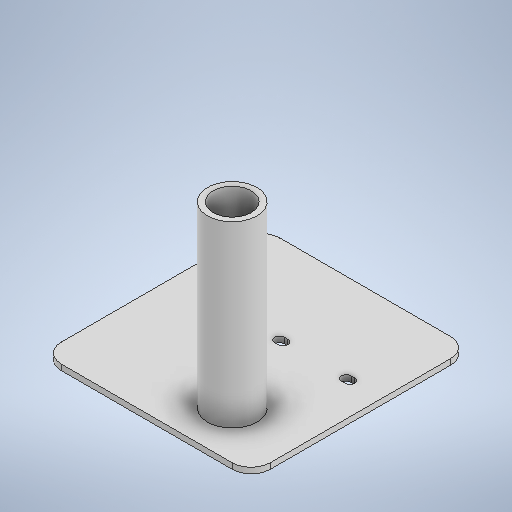
# Autodesk Inventor part: TopMount
Saved by Autodesk Inventor 2025.2 (Build 292293000, 293)
## iProperties
Created: 2025-07-18
Part Number: TopMount
Material: Generic
Document SubType Name: Modeling
Designer: Simon
Density: 1 g/cm^3
Appearance: Default
Author: Simon
Autodesk Inventor part; units mm, degrees
ref_plane "YZ Plane" through (0, 0, 0) normal (1, 0, 0) x (0, 1, 0)
ref_plane "XZ Plane" through (0, 0, 0) normal (0, 1, 0) x (-1, 0, 0)
ref_plane "XY Plane" through (0, 0, 0) normal (0, 0, 1) x (1, 0, 0)
sketch "Sketch1" plane through (0, 0, 0) normal (0, 1, 0) x (-1, 0, 0)
  line L0 (-75, 47.5) -> (75, 47.5)
  line L1 (75, 47.5) -> (75, -47.5)
  line L2 (75, -47.5) -> (-75, -47.5)
  line L3 (-75, -47.5) -> (-75, 47.5)
  line L4 (-75, 47.5) -> (75, -47.5) construction
  line L5 (75, 47.5) -> (-75, -47.5) construction
  point P0 (0, 0)
  dimension "d0" = 150
  dimension "d1" = 95
  constraints: 12 end point, 2 midpoint, 2 parallel, 1 horizontal, 1 perpendicular
  measures "d0" distance of L1.end L2.end
  measures "d1" distance of L0.end L1.end
extrude "Extrusion1" add sketch "Sketch1" along normal blind 3
sketch "Sketch6" plane through (0, 3, 0) normal (0, 1, 0) x (1, 0, 0)
  line L0 (75, 47.5) -> (-75, 47.5) projected
  line L1 (0, 47.5) -> (0, 22.5)
  line L2 (0, 22.5) -> (0, -20.7)
  line L3 (0, -20.7) -> (0, 0.9)
  line L4 (0, 0.9) -> (-53.4, 0.9)
  line L5 (-18.65, 0.9) -> (18.65, 0.9)
  circle A0 centre (18.65, 0.9) radius 2.5
  circle A1 centre (-18.65, 0.9) radius 2.5
  line L6 (-18.65, 0.9) -> (-16.65, 0.9)
  line L7 (18.65, 0.9) -> (16.65, 0.9)
  circle A2 centre (16.65, 0.9) radius 2.5
  circle A3 centre (-16.65, 0.9) radius 2.5
  line L8 (-18.65, 3.4) -> (-16.65, 3.4)
  line L9 (-18.65, -1.6) -> (-16.65, -1.6)
  line L10 (16.65, 3.4) -> (18.65, 3.4)
  line L11 (16.65, -1.6) -> (18.65, -1.6)
  point P0 (0, 0)
  dimension "d40" = 25
  dimension "d41" = 43.2
  dimension "d42" = 53.4
  dimension "d46" = 37.3
  dimension "d47" = 5
  dimension "d48" = 5
  dimension "d49" = 2
  dimension "d50" = 2
  dimension "d51" = 5
  dimension "d52" = 5
  constraints: 22 end point, 8 point on circle, 8 tangent, 4 centre point, 4 coincident, 3 midpoint, 3 point on line, 1 horizontal, 1 perpendicular, 1 vertical
  measures "d40" distance of L1.start L1.end
  measures "d41" distance of L1.end L2.end
  measures "d42" distance of L3.end L4.end
  measures "d46" distance of L5.start L5.end
  measures "d47" diameter of A0
  measures "d48" diameter of A1
  measures "d49" distance of L6.start L6.end
  measures "d50" distance of L7.start L7.end
  measures "d51" diameter of A2
  measures "d52" diameter of A3
extrude "Extrusion6" cut sketch "Sketch6" against normal through all
sketch "Sketch7" plane through (0, 3, 0) normal (0, 1, 0) x (1, 0, 0)
  line L0 (75, 47.5) -> (-75, 47.5) projected
  line L1 (-75, -47.5) -> (75, -47.5) projected
  line L2 (75, 47.5) -> (35, 47.5)
  line L3 (35, 47.5) -> (35, -47.5)
  line L4 (35, -47.5) -> (75, -47.5)
  line L5 (75, -47.5) -> (75, 47.5)
  point P0 (0, 0)
  point P1 (75, -47.5)
  dimension "d55" = 40
  constraints: 8 end point, 2 parallel, 1 horizontal, 1 perpendicular, 1 point on line
  measures "d55" distance of L4.end L3.end
extrude "Extrusion7" cut sketch "Sketch7" against normal through all
sketch "Sketch8" plane through (0, 3, 0) normal (0, 1, 0) x (1, 0, 0)
  line L0 (-75, -47.5) -> (35, -47.5) projected
  line L1 (35, 47.5) -> (-75, 47.5) projected
  line L2 (0, 47.5) -> (0, -42.5)
  circle A0 centre (0, -42.5) radius 13
  line L3 (0, -42.5) -> (-20, -42.5)
  circle A1 centre (-20, -42.5) radius 1.5
  circle A2 centre (-10, -59.8205) radius 1.5
  circle A3 centre (10, -59.8205) radius 1.5
  circle A4 centre (20, -42.5) radius 1.5
  circle A5 centre (10, -25.1795) radius 1.5
  circle A6 centre (-10, -25.1795) radius 1.5
  circle A7 centre (0, -42.5) radius 10
  point P0 (0, 0)
  point P1 (7, 47.5)
  point P2 (-7, 47.5)
  point P3 (-10, -42.5)
  point P4 (-10, -47.5)
  point P5 (10, -42.5)
  point P6 (10, -47.5)
  point P7 (8.6603, -47.5)
  point P8 (-8.6603, -47.5)
  dimension "d60" = 90
  dimension "d62" = 26
  dimension "d63" = 20
  dimension "d64" = 3
  dimension "d67" = 360
  dimension "d69" = 20
  constraints: 8 centre point, 7 coincident, 4 end point, 3 point on line, 2 point on circle, 1 horizontal, 1 perpendicular, 19 other
  measures "d60" distance of L2.start L2.end
  measures "d62" diameter of A0
  measures "d63" distance of L3.start L3.end
  measures "d64" diameter of A1
  measures "d69" diameter of A7
sketch "Sketch9" plane through (-75, 0, 47.5) normal (0, 0, 1) x (1, 0, 0)
  line L0 (110, 0) -> (0, 0) projected
  line L1 (110, 3) -> (110, 0) projected
  line L2 (0, 0) -> (110, 0)
  line L3 (110, 0) -> (110, 3)
  line L4 (110, 3) -> (0, 3)
  line L5 (0, 3) -> (0, 0)
  point P0 (75, 0)
  constraints: 8 end point, 2 parallel, 1 horizontal, 1 perpendicular
extrude "Extrusion9" add sketch "Sketch9" along normal blind 20
extrude "Extrusion10" add sketch "Sketch8" along normal blind 94 contours A0 L3 A7 L0 | L0 A7 A0 | A0 L2 A7 L3 | L0 A7 L2 A0
sketch "Sketch10" plane through (0, 3, 42.5) normal (0, 1, 0) x (1, 0, 0)
  circle A0 centre (0, 0) radius 1
  point P0 (0, 42.5)
  dimension "d77" = 2
  constraints: 1 centre point
  measures "d77" diameter of A0
extrude "Extrusion11" cut sketch "Sketch10" against normal through all
sketch "Sketch11" plane through (0, 0, 0) normal (0, -1, 0) x (1, 0, 0)
  circle A0 centre (0, 42.5) radius 1 projected
  circle A1 centre (0, 42.5) radius 1
  circle A2 centre (0, 42.5) radius 2
  point P0 (0, 0)
  dimension "d80" = 4
  constraints: 2 centre point, 2 coincident
  measures "d80" diameter of A2
extrude "Extrusion12" add sketch "Sketch11" along normal blind 5
thread "Thread1" size "M4x0.7" class "6g" standard "ISO Metric profile" full length
fillet "Fillet2" radius 10 4 edges at (35, 1.5, 67.5) (35, 1.5, -47.5) (-75, 1.5, 67.5) (-75, 1.5, -47.5)
body "Solid1"
